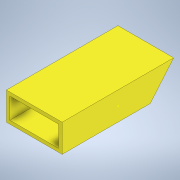
# Autodesk Inventor part: Aluminum1x2HypotTop
Saved by Autodesk Inventor 2020.2 (Build 242310000, 310)
## iProperties
Created: 2020-01-26
Part Number: Aluminum1x2HypotTop
Material: Aluminum 6061
Document SubType Name: Modeling
Designer: robst
Density: 2.7 g/cm^3
Appearance: Canary
Author: robst
Autodesk Inventor part; units mm, degrees
ref_plane "YZ Plane" through (0, 0, 0) normal (1, 0, 0) x (0, 1, 0)
ref_plane "XZ Plane" through (0, 0, 0) normal (0, 1, 0) x (-1, 0, 0)
ref_plane "XY Plane" through (0, 0, 0) normal (0, 0, 1) x (1, 0, 0)
sketch "Sketch1" plane through (0, 0, 0) normal (0, 0, 1) x (1, 0, 0)
  line L0 (-25.4, -12.7) -> (25.4, -12.7)
  line L1 (25.4, -12.7) -> (25.4, 12.7)
  line L2 (25.4, 12.7) -> (-25.4, 12.7)
  line L3 (-25.4, 12.7) -> (-25.4, -12.7)
  line L4 (-25.4, -12.7) -> (25.4, 12.7) construction
  line L5 (25.4, -12.7) -> (-25.4, 12.7) construction
  line L6 (-22.225, -9.525) -> (22.225, -9.525)
  line L7 (22.225, -9.525) -> (22.225, 9.525)
  line L8 (22.225, 9.525) -> (-22.225, 9.525)
  line L9 (-22.225, 9.525) -> (-22.225, -9.525)
  line L10 (-22.225, -9.525) -> (22.225, 9.525) construction
  line L11 (22.225, -9.525) -> (-22.225, 9.525) construction
  point P0 (0, 0)
  dimension "d0" = 50.8
  dimension "d1" = 25.4
  dimension "d2" = 3.175
  dimension "d3" = 3.175
  constraints: 24 end point, 5 parallel, 4 midpoint, 2 perpendicular, 1 horizontal
  measures "d0" distance of L0.start L0.end
  measures "d1" distance of L1.end L0.end
  measures "d2" distance between parallel lines of L0 L6
  measures "d3" distance between parallel lines of L3 L9
extrude "Extrusion1" add sketch "Sketch1" along normal mid plane 101.6
sketch "Sketch2" plane through (25.4, -12.7, 50.8) normal (1, 0, 0) x (0, 0, -1)
  point P0 (50.8, 12.7)
sketch "Sketch3" plane through (25.4, -12.7, 50.8) normal (1, 0, 0) x (0, 0, -1)
  line L0 (101.6, 0) -> (101.6, 25.4) projected
  line L1 (101.6, 25.4) -> (80.2869, 0)
  line L2 (101.6, 0) -> (0, 0) projected
  line L3 (101.6, 25.4) -> (101.6, 0)
  line L4 (101.6, 3.175) -> (101.6, 22.225) projected
  line L5 (101.6, 0) -> (80.2869, 0)
  point P0 (50.8, 12.7)
  dimension "d6" = 50
  constraints: 6 end point, 1 collinear, 1 perpendicular, 1 point on line
  measures "d6" angle of L1 L2
extrude "Extrusion2" cut sketch "Sketch3" against normal through all
body "Solid1"
